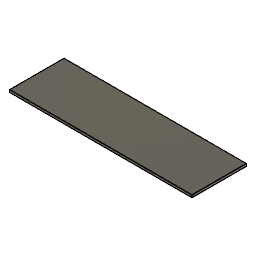
Canal - top plate v1 (Autodesk Fusion 360 design; units mm, degrees)
Autodesk Fusion 360 part; units mm, degrees
sketch "Esquisse1" plane through (0, 0, 0) normal (0, 0, 1) x (1, 0, 0)
  line L0 (-5.6946, 30) -> (67.3054, 30)
  line L1 (67.3054, 30) -> (67.3054, 8.2)
  line L2 (67.3054, 8.2) -> (-5.6946, 8.2)
  line L3 (-5.6946, 8.2) -> (-5.6946, 30)
  dimension "d1" = 73
  dimension "d2" = 21.8
  constraint horizontal L0
  constraint vertical L1
  constraint horizontal L2
  constraint vertical L3
  measures "d1" distance of L1 L3
  measures "d2" distance of L0 L2
extrude "Extrusion1" add sketch "Esquisse1" along normal blind 1
